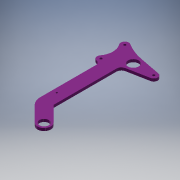
# Autodesk Inventor part: Intake Arms
Saved by Autodesk Inventor 2017 (Build 210142000, 142)
## iProperties
Created: 2017-01-12
Part Number: Intake Arms
Material: Generic
Document SubType Name: Modeling
Designer: Ben
Density: 1 g/cm^3
Appearance: Smooth - Purple
Author: Ben
Autodesk Inventor part; units mm, degrees
ref_plane "YZ Plane" through (0, 0, 0) normal (1, 0, 0) x (0, 1, 0)
ref_plane "XZ Plane" through (0, 0, 0) normal (0, 1, 0) x (-1, 0, 0)
ref_plane "XY Plane" through (0, 0, 0) normal (0, 0, 1) x (1, 0, 0)
sketch "Sketch1" plane through (0, 0, 0) normal (0, 1, 0) x (-1, 0, 0)
  circle A0 centre (0, 0) radius 11.1125
  line L0 (0, -228.6) -> (0, 0) construction
  line L1 (15.875, -228.6) -> (0, -228.6) construction
  circle A1 centre (15.875, -228.6) radius 12.7
  line L2 (25.4, -47.8506) -> (25.4, -198.0228)
  line L3 (57.15, -47.8506) -> (57.15, -181.2924)
  arc A2 (11.2253, 11.2253) -> (-11.2253, -11.2253) centre (0, 0) ccw
  line L4 (-11.2253, -11.2253) -> (25.4, -47.8506)
  arc A3 (57.15, -47.8506) -> (47.8506, -25.4) centre (25.4, -47.8506) ccw
  line L5 (47.8506, -25.4) -> (11.2253, 11.2253)
  circle A4 centre (64.5922, -200.2282) radius 2.8067
  circle A5 centre (64.5922, -256.9718) radius 2.8067
  line L6 (64.5922, -256.9718) -> (64.5922, -200.2282) construction
  line L7 (15.875, -228.6) -> (64.5922, -228.6) construction
  line L8 (15.875, -228.6) -> (-32.8422, -228.6) construction
  circle A6 centre (-32.8422, -228.6) radius 2.8067
  arc A7 (-34.6377, -219.2458) -> (-34.6377, -237.9542) centre (-32.8422, -228.6) ccw
  arc A8 (59.4685, -265.0013) -> (72.1876, -251.2241) centre (64.5922, -256.9718) ccw
  arc A9 (72.1876, -205.9759) -> (65.6336, -190.7603) centre (64.5922, -200.2282) ccw
  line L9 (15.875, -247.65) -> (-34.6377, -237.9542)
  line L10 (15.875, -247.65) -> (15.875, -228.6) construction
  arc A10 (59.4685, -265.0013) -> (15.875, -247.65) centre (-7.6434, -370.1755) ccw
  arc A11 (72.1876, -205.9759) -> (72.1876, -251.2241) centre (102.0848, -228.6) ccw
  arc A12 (57.15, -181.2924) -> (65.6336, -190.7603) centre (66.675, -181.2924) ccw
  line L11 (-34.6377, -219.2458) -> (15.875, -209.55)
  arc A13 (15.875, -209.55) -> (25.4, -198.0228) centre (13.6624, -198.0228) ccw
  line L12 (15.875, -228.6) -> (15.875, -209.55) construction
  line L13 (15.875, -228.6) -> (0, 0) construction
  line L14 (5.5429, -79.8178) -> (46.7187, -76.9583) construction
  circle A14 centre (46.7187, -76.9583) radius 1.905
  dimension "d0" = 22.225
  dimension "d2" = 228.6
  dimension "d7" = 25.4
  dimension "d17" = 31.75
  dimension "d18" = 45
  dimension "d20" = 25.4
  dimension "d21" = 56.7436
  dimension "d22" = 5.6134
  dimension "d23" = 48.7172
  dimension "d24" = 48.7172
  dimension "d25" = 9.525
  dimension "d26" = 19.05
  dimension "d27" = 19.05
  dimension "d28" = 15.875
  dimension "d29" = 3.81
  dimension "d31" = 41.275
  dimension "d32" = 80.01
  constraints: 31 end point, 18 point on circle, 15 centre point, 15 tangent, 8 coincident, 6 vertical, 5 equal radius, 3 horizontal, 1 midpoint, 1 parallel, 1 perpendicular, 1 point on line
  measures "d0" diameter of A0
  measures "d2" distance of point (0, 0) L0.start
  measures "d7" diameter of A1
  measures "d17" diameter of A2
  measures "d18" angle of L2 L4
  measures "d20" distance between parallel lines of L0 L2
  measures "d21" distance of L6.start L6.end
  measures "d22" diameter of A5
  measures "d23" distance of L1.start L7.end
  measures "d24" distance of L1.start L8.end
  measures "d25" radius of A7
  measures "d26" distance of L9.start L1.start
  measures "d27" distance of L1.start L11.end
  measures "d28" distance from line of L0 L1.start
  measures "d29" diameter of A14
  measures "d31" distance of L14.start L14.end
  measures "d32" distance of point (0, 0) L14.start
extrude "Extrusion1" add sketch "Sketch1" along normal blind 6.35
equation "\"d24\" = d23"
equation "\"d27\" = d26"
body "Solid1"
